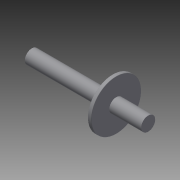
# Autodesk Inventor part: axlie
Saved by Autodesk Inventor 2015 (Build 190159000, 159)
## iProperties
Created: 2015-09-29
Part Number: axlie
Material: Generic
Document SubType Name: Modeling
Designer: Ross
Density: 1 g/cm^3
Appearance: Default
Author: Ross
Autodesk Inventor part; units mm, degrees
ref_plane "YZ Plane" through (0, 0, 0) normal (1, 0, 0) x (0, 1, 0)
ref_plane "XZ Plane" through (0, 0, 0) normal (0, 1, 0) x (-1, 0, 0)
ref_plane "XY Plane" through (0, 0, 0) normal (0, 0, 1) x (1, 0, 0)
sketch "Sketch1" plane through (0, 0, 0) normal (0, 0, 1) x (1, 0, 0)
  line L0 (0, 0) -> (0, 3.9)
  line L1 (0, 3.9) -> (-17.7557, 3.9)
  line L2 (-17.7557, 3.9) -> (-2.7557, 3.9)
  line L3 (-17.7557, 3.9) -> (-17.7557, 13.9)
  line L4 (-17.7557, 13.9) -> (-19.7557, 13.9)
  line L5 (-19.7557, 13.9) -> (-19.7557, 3.9)
  line L6 (-19.7557, 3.9) -> (-34.7557, 3.9)
  line L7 (-34.7557, 3.9) -> (-64.7557, 3.9)
  line L8 (-64.7557, 3.9) -> (-64.7557, 0)
  line L9 (-64.7557, 0) -> (0, 0)
  dimension "d0" = 3.9
  dimension "d1" = 15
  dimension "d2" = 10
  dimension "d3" = 2
  dimension "d4" = 10
  dimension "d5" = 15
  dimension "d6" = 30
  constraints: 20 end point, 6 perpendicular, 2 vertical, 1 horizontal, 1 point on line
  measures "d0" distance of L0.start L0.end
  measures "d1" distance of L1.end L2.end
  measures "d2" distance of L1.end L3.end
  measures "d3" distance of L3.end L4.end
  measures "d4" distance of L4.end L5.end
  measures "d5" distance of L5.end L6.end
  measures "d6" distance of L6.end L7.end
revolve "Revolution1" add sketch "Sketch1" angle 360 about axis through (-64.7557, 0, 0) along (1, 0, 0)
fillet "Fillet1" radius 0.2 2 edges at (-19.7557, -13.9, 0) (-17.7557, -13.9, 0)
body "Solid1"
